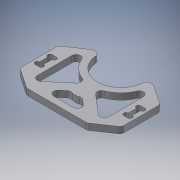
# Autodesk Inventor part: 付け根_メインフレーム_6_1
Saved by Autodesk Inventor 2018 (Build 220112000, 112)
## iProperties
Created: 2016-08-24
Part Number: 付け根_メインフレーム_6_1
Material: アルミニウム 2014-T4
Document SubType Name: Modeling
Designer: hiro
Density: 2.8 g/cm^3
Appearance: サテン
Mass: 5.61362 g
Surface Area: 25.3587 cm^2
Volume: 2.00486 cm^3
Author: hiro
Autodesk Inventor part; units mm, degrees
ref_plane "YZ Plane" through (0, 0, 0) normal (1, 0, 0) x (0, 1, 0)
ref_plane "XZ Plane" through (0, 0, 0) normal (0, 1, 0) x (-1, 0, 0)
ref_plane "XY Plane" through (0, 0, 0) normal (0, 0, 1) x (1, 0, 0)
derived "付け根_基準フレーム_6_1.ipt"
sketch "スケッチ1" plane through (0, 0, 0) normal (0, 0, 1) x (1, 0, 0)
  circle A0 centre (0, 0) radius 11 construction
  circle A1 centre (-13.5, -1) radius 1.35
  line L0 (-13.5, -1) -> (13.5, -1) construction
  line L1 (13.5, -1) -> (13.5, -28) construction
  line L2 (13.5, -28) -> (-13.5, -28) construction
  line L3 (-13.5, -28) -> (-13.5, -1) construction
  circle A2 centre (13.5, -1) radius 1.35
  circle A3 centre (-13.5, -28) radius 1.35
  circle A4 centre (13.5, -28) radius 1.35
  line L4 (0, 16.5) -> (0, -16.5) construction
  circle A5 centre (0, -16.5) radius 5.5 construction
  line L5 (-12.5, 27) -> (-12.5, 22) construction
  line L6 (-12.5, 22) -> (-5.9183, -17.4865) construction
  line L7 (-12.5, 27) -> (12.5, 27) construction
  line L8 (12.5, 27) -> (12.5, 22) construction
  line L9 (12.5, 22) -> (5.9183, -17.4865) construction
  arc A6 (-5.9183, -17.4865) -> (5.9183, -17.4865) centre (0, -16.5) ccw construction
  circle A7 centre (-9.5, 24.5) radius 1.55 construction
  circle A8 centre (9.5, 24.5) radius 1.55 construction
  line L10 (-5.55, 24.55) -> (5.55, 24.55) construction
  line L11 (5.55, 24.55) -> (5.55, 21.95) construction
  line L12 (5.55, 21.95) -> (-5.55, 21.95) construction
  line L13 (-5.55, 21.95) -> (-5.55, 24.55) construction
  circle A9 centre (-4.5, 24.55) radius 1.05 construction
  circle A10 centre (-4.5, 21.95) radius 1.05 construction
  circle A11 centre (4.5, 24.55) radius 1.05 construction
  circle A12 centre (4.5, 21.95) radius 1.05 construction
  line L14 (5.5, 24.5) -> (-5.5, 24.5) construction
  line L15 (-5.5, 24.5) -> (-5.5, 22) construction
  line L16 (-5.5, 22) -> (5.5, 22) construction
  line L17 (5.5, 22) -> (5.5, 24.5) construction
  circle A13 centre (0, -16.5) radius 4.05 construction
  circle A14 centre (0, 8.5) radius 1.35 construction
  circle A15 centre (-8.5, 0) radius 1.35 construction
  circle A16 centre (0, -8.5) radius 1.35 construction
  circle A17 centre (8.5, 0) radius 1.35 construction
  circle A18 centre (0, 0) radius 5.05 construction
  line L18 (-9.7809, 5.0333) -> (-3.0676, 18.0786) construction
  line L19 (3.0676, 18.0786) -> (9.7809, 5.0333) construction
  arc A19 (-9.7809, 5.0333) -> (9.7809, 5.0333) centre (0, 0) ccw construction
  arc A20 (3.0676, 18.0786) -> (-3.0676, 18.0786) centre (0, 16.5) ccw construction
  circle A21 centre (0, 16.5) radius 1.55 construction
  line L20 (-10.9545, 1) -> (-14.1083, 1)
  line L21 (-14.1083, 1) -> (-23.805, -5.5)
  line L22 (-23.805, -5.5) -> (-23.805, -23.5)
  line L23 (-23.805, -23.5) -> (-14.1083, -30)
  line L24 (-14.1083, -30) -> (14.1083, -30)
  line L25 (14.1083, -30) -> (23.805, -23.5)
  line L26 (23.805, -23.5) -> (23.805, -5.5)
  line L27 (23.805, -5.5) -> (14.1083, 1)
  line L28 (14.1083, 1) -> (10.9545, 1)
  arc A22 (-10.9545, 1) -> (10.9545, 1) centre (0, 0) ccw
  line L29 (-21.755, -10.495) -> (-19.745, -10.495)
  line L30 (-19.745, -10.495) -> (-19.745, -18.505)
  line L31 (-19.745, -18.505) -> (-21.755, -18.505)
  line L32 (-21.755, -18.505) -> (-21.755, -10.495)
  line L33 (-19.75, -10.5) -> (-21.75, -10.5) construction
  line L34 (-21.75, -10.5) -> (-21.75, -18.5) construction
  line L35 (-21.75, -18.5) -> (-19.75, -18.5) construction
  line L36 (-19.75, -18.5) -> (-19.75, -10.5) construction
  circle A23 centre (-21.755, -11.545) radius 1.05
  circle A24 centre (-19.745, -11.545) radius 1.05
  circle A25 centre (-19.745, -17.455) radius 1.05
  circle A26 centre (-21.755, -17.455) radius 1.05
  circle A27 centre (-13.5, -1) radius 2 construction
  line L37 (-23.805, -14.5) -> (-19.75, -14.5) construction
  circle A28 centre (-21.755, -11.545) radius 2.05 construction
  circle A29 centre (-13.5, -28) radius 2 construction
  line L38 (21.755, -10.495) -> (19.745, -10.495)
  line L39 (19.75, -10.5) -> (21.75, -10.5) construction
  circle A30 centre (19.745, -11.545) radius 1.05
  circle A31 centre (21.755, -11.545) radius 1.05
  circle A32 centre (21.755, -11.545) radius 2.05 construction
  line L40 (23.805, -14.5) -> (19.75, -14.5) construction
  line L41 (19.75, -18.5) -> (19.75, -10.5) construction
  line L42 (21.75, -10.5) -> (21.75, -18.5) construction
  line L43 (19.745, -10.495) -> (19.745, -18.505)
  line L44 (21.755, -18.505) -> (21.755, -10.495)
  circle A33 centre (19.745, -17.455) radius 1.05
  line L45 (21.75, -18.5) -> (19.75, -18.5) construction
  line L46 (19.745, -18.505) -> (21.755, -18.505)
  circle A34 centre (21.755, -17.455) radius 1.05
  line L47 (0, -13.2668) -> (2.8, -14.8834) construction
  line L48 (2.8, -14.8834) -> (2.8, -18.1166) construction
  line L49 (2.8, -18.1166) -> (0, -19.7332) construction
  line L50 (0, -19.7332) -> (-2.8, -18.1166) construction
  line L51 (-2.8, -18.1166) -> (-2.8, -14.8834) construction
  line L52 (-2.8, -14.8834) -> (0, -13.2668) construction
  line L53 (-19.75, 12) -> (19.75, 12) construction
  line L54 (19.75, 12) -> (19.75, -39.5) construction
  line L55 (19.75, -39.5) -> (-19.75, -39.5) construction
  line L56 (-19.75, -39.5) -> (-19.75, 12) construction
  arc A35 (3.5, 16.5) -> (-3.5, 16.5) centre (0, 16.5) ccw construction
  line L57 (-3.5, 16.5) -> (-3.5, 6.8345) construction
  line L58 (3.5, 16.5) -> (3.5, 6.8345) construction
  arc A36 (-3.5, 6.8345) -> (3.5, 6.8345) centre (0, 6.8345) ccw construction
  circle A37 centre (0, 16.5) radius 5.5 construction
  circle A38 centre (0, -16.5) radius 1.55
  line L59 (-21.75, -2) -> (-19.75, -2) construction
  line L60 (-19.75, -2) -> (-19.75, -27) construction
  line L61 (-19.75, -27) -> (-21.75, -27) construction
  line L62 (-21.75, -27) -> (-21.75, -2) construction
  circle A39 centre (0, -16.5) radius 33 construction
  line L63 (0, -16.5) -> (-23.3345, 6.8345) construction
  circle A40 centre (0, 0) radius 16.5 construction
  line L64 (-16.5, 0) -> (-23.3345, 6.8345) construction
  point P0 (0, -1)
  point P1 (0, 27)
  point P2 (-12.5, 24.5)
  point P3 (-21.75, -14.5)
  dimension "d1" = 3.1
  measures "d1" diameter of A38
extrude "押し出し1" add sketch "スケッチ1" along normal blind 3
sketch "スケッチ4" plane through (0, 0, 3) normal (0, 0, 1) x (1, 0, 0)
  line L0 (-19.745, -18.505) -> (-21.755, -18.505) projected
  arc A0 (-21.755, -16.405) -> (-21.755, -18.505) centre (-21.755, -17.455) ccw projected
  line L1 (-21.755, -16.405) -> (-21.755, -12.595) projected
  arc A1 (-21.755, -10.495) -> (-21.755, -12.595) centre (-21.755, -11.545) ccw projected
  line L2 (-21.755, -10.495) -> (-19.745, -10.495) projected
  arc A2 (-19.745, -12.595) -> (-19.745, -10.495) centre (-19.745, -11.545) ccw projected
  line L3 (-19.745, -12.595) -> (-19.745, -16.405) projected
  arc A3 (-19.745, -18.505) -> (-19.745, -16.405) centre (-19.745, -17.455) ccw projected
  circle A4 centre (0, -16.5) radius 1.55 projected
  circle A5 centre (13.5, -28) radius 1.35 projected
  circle A6 centre (-13.5, -28) radius 1.35 projected
  circle A7 centre (-13.5, -1) radius 1.35 projected
  line L4 (-14.1083, -30) -> (14.1083, -30) projected
  arc A8 (-10.9545, 1) -> (10.9545, 1) centre (0, 0) ccw projected
  line L5 (-10.0129, -27) -> (10.0129, -27)
  line L6 (10.0129, -27) -> (2.6582, -20.7349)
  line L7 (-10.0129, -27) -> (-2.6582, -20.7349)
  arc A9 (-2.6582, -20.7349) -> (2.6582, -20.7349) centre (0, -16.5) ccw
  line L8 (0, -16.5) -> (-13.5, -28) construction
  line L9 (0, -16.5) -> (13.5, -28) construction
  line L10 (-16.75, -4) -> (-16.75, -26.8276)
  line L11 (-16.75, -26.8276) -> (-3, -15.1146)
  line L12 (-16.75, -4) -> (-13.4164, -4)
  arc A10 (-13.4164, -4) -> (-3, -13.6748) centre (0, 0) ccw
  line L13 (-19.745, -10.5) -> (-21.755, -10.5) construction
  arc A11 (-21.755, -10.5) -> (-21.75, -12.59) centre (-21.755, -11.545) ccw construction
  line L14 (-21.75, -12.59) -> (-21.75, -16.41) construction
  arc A12 (-21.75, -16.41) -> (-21.755, -18.5) centre (-21.755, -17.455) ccw construction
  line L15 (-21.755, -18.5) -> (-19.745, -18.5) construction
  arc A13 (-19.745, -18.5) -> (-19.75, -16.41) centre (-19.745, -17.455) ccw construction
  line L16 (-19.75, -16.41) -> (-19.75, -12.59) construction
  arc A14 (-19.75, -12.59) -> (-19.745, -10.5) centre (-19.745, -11.545) ccw construction
  line L17 (0, 0) -> (0, -16.5) construction
  line L18 (16.75, -4) -> (16.75, -26.8276)
  line L19 (16.75, -26.8276) -> (3, -15.1146)
  line L20 (16.75, -4) -> (13.4164, -4)
  arc A15 (3, -13.6748) -> (13.4164, -4) centre (0, 0) ccw
  line L21 (-3, -13.6748) -> (-3, -15.1146)
  line L22 (3, -13.6748) -> (3, -15.1146)
  dimension "d13" = 5
  dimension "d14" = 3
  dimension "d15" = 1.5
  dimension "d16" = 3
  dimension "d17" = 3
  dimension "d18" = 0.005
  dimension "d19" = 3
  dimension "d20" = 3
  dimension "d24" = 3
  constraints: 36 end point, 14 point on circle, 7 centre point, 4 symmetric about line, 3 parallel, 3 vertical, 2 coincident, 2 equal length, 2 horizontal, 8 other
  measures "d13" radius of A9
  measures "d14" distance between parallel lines of L5 L4
  measures "d15" distance between parallel lines of L8 L7
  measures "d16" radial gap between concentric circles of A8 A10
  measures "d17" distance between parallel lines of L8 L11
  measures "d18" distance between parallel lines of L2 L13
  measures "d19" distance between parallel lines of L10 L16
  measures "d20" distance from line of A7.centre L12
  measures "d24" distance between parallel lines of L17 L21
extrude "押し出し3" cut sketch "スケッチ4" against normal blind 3 contours L7 A9 L6 L5 | L12 A10 L21 L11 L10 | L18 L19 L22 A15 L20
fillet "フィレット2" radius 2 24 edges at (-16.75, -4, 1.5) (-13.4164, -4, 1.5) (-10.9545, 1, 1.5) (-14.1083, 1, 1.5) (-23.805, -5.5, 1.5) (-23.805, -23.5, 1.5) (-16.75, -26.8276, 1.5) (-3, -13.6748, 1.5) (3, -13.6748, 1.5) (10.9545, 1, 1.5) (14.1083, 1, 1.5) (16.75, -4, 1.5) (13.4164, -4, 1.5) (23.805, -5.5, 1.5) (23.805, -23.5, 1.5) (16.75, -26.8276, 1.5) (14.1083, -30, 1.5) (-14.1083, -30, 1.5) (-10.0129, -27, 1.5) (-2.6582, -20.7349, 1.5) (2.6582, -20.7349, 1.5) (10.0129, -27, 1.5) (3, -15.1146, 1.5) (-3, -15.1146, 1.5)
sketch "スケッチ5" plane through (0, 0, 3) normal (0, 0, 1) x (1, 0, 0)
  circle A0 centre (-13.5, -1) radius 1.35 projected
  circle A1 centre (-13.5, -1) radius 1.35
  circle A2 centre (0, -16.5) radius 1.55 projected
  circle A3 centre (0, -16.5) radius 1.55
  circle A4 centre (-13.5, -28) radius 1.35 projected
  circle A5 centre (-13.5, -28) radius 1.35
  circle A6 centre (13.5, -28) radius 1.35 projected
  circle A7 centre (13.5, -28) radius 1.35
  circle A8 centre (13.5, -1) radius 1.35 projected
  circle A9 centre (13.5, -1) radius 1.35
  point P0 (0, 0)
  constraints: 5 centre point, 5 coincident
extrude "押し出し4" add sketch "スケッチ5" against normal up to surface (3 mm away)
